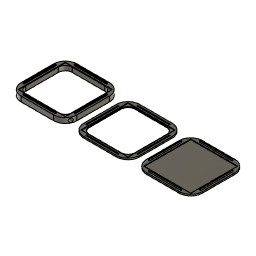
Abyssal_Mirror (Autodesk Fusion 360 design; units mm, degrees)
Autodesk Fusion 360 part; units mm, degrees
sketch "草图1" plane through (0, 0, 0) normal (0, 0, 1) x (1, 0, 0)
  line L0 (-50.5, 50.5) -> (50.5, 50.5)
  line L1 (50.5, 50.5) -> (50.5, -50.5)
  line L2 (50.5, -50.5) -> (-50.5, -50.5)
  line L3 (-50.5, -50.5) -> (-50.5, 50.5)
  line L4 (-35, 50) -> (35, 50)
  line L5 (50, 35) -> (50, -35)
  line L6 (35, -50) -> (-35, -50)
  line L7 (-50, -35) -> (-50, 35)
  arc A0 (-35, 50) -> (-50, 35) centre (-35, 35) ccw
  arc A1 (50, 35) -> (35, 50) centre (35, 35) ccw
  arc A2 (35, -50) -> (50, -35) centre (35, -35) ccw
  arc A3 (-50, -35) -> (-35, -50) centre (-35, -35) ccw
  line L8 (-35, 60) -> (35, 60)
  line L9 (60, 35) -> (60, -35)
  line L10 (35, -60) -> (-35, -60)
  line L11 (-60, -35) -> (-60, 35)
  arc A4 (60, 35) -> (35, 60) centre (35, 35) ccw
  arc A5 (-35, 60) -> (-60, 35) centre (-35, 35) ccw
  arc A6 (-60, -35) -> (-35, -60) centre (-35, -35) ccw
  arc A7 (35, -60) -> (60, -35) centre (35, -35) ccw
  dimension "d1" = 101
  dimension "d2" = 101
  dimension "d3" = 15
  dimension "d4" = 15
  dimension "d5" = 25
  constraint horizontal L0
  constraint vertical L1
  constraint horizontal L2
  constraint vertical L3
  constraint horizontal L4
  constraint vertical L5
  constraint horizontal L6
  constraint vertical L7
  constraint tangent L4 A0
  constraint tangent L7 A0
  constraint tangent L4 A1
  constraint tangent L5 A1
  constraint tangent L5 A2
  constraint tangent L6 A2
  constraint equal A1 A2
  constraint tangent L7 A3
  constraint tangent L6 A3
  constraint equal A1 A3
  constraint horizontal L8
  constraint vertical L9
  constraint horizontal L10
  constraint vertical L11
  constraint tangent L9 A4
  constraint tangent L8 A4
  constraint tangent L8 A5
  constraint tangent L11 A5
  constraint equal A4 A5
  constraint tangent L11 A6
  constraint tangent L10 A6
  constraint equal A4 A6
  constraint tangent L9 A7
  constraint tangent L10 A7
  constraint equal A4 A7
  measures "d1" distance of L0.start L0.end
  measures "d2" distance of L0.start L2.end
  measures "d3" radius of A0
  measures "d4" radius of A1
  measures "d5" radius of A4
extrude "拉伸1" add sketch "草图1" along normal blind 11 contours L8 L9 L10 L11 A4 A5 A6 A7 makes body 1
extrude "拉伸2" add sketch "草图1" along normal blind 9 contours L0 L1 L2 L3 bodies 1
sketch "草图2" plane through (0, 0, 0) normal (0, 0, 1) x (1, 0, 0)
  line L0 (-35, 56) -> (35, 56)
  line L1 (35, 56) -> (35, 54)
  line L2 (35, 54) -> (-35, 54)
  line L3 (-35, 54) -> (-35, 56)
  line L4 (53.9983, 35) -> (56, 35)
  line L5 (56, 35) -> (56, -35)
  line L6 (56, -35) -> (53.9983, -35)
  line L7 (53.9983, -35) -> (53.9983, 35)
  line L8 (-5, 0) -> (5, 0)
  line L9 (0, 5) -> (0, -5)
  line L10 (35, -56) -> (35, -54)
  line L11 (-35, -54) -> (-35, -56)
  line L12 (-35, -56) -> (35, -56)
  line L13 (35, -54) -> (-35, -54)
  line L14 (-56, -35) -> (-53.9983, -35)
  line L15 (-56, 35) -> (-56, -35)
  line L16 (-53.9983, -35) -> (-53.9983, 35)
  line L17 (-53.9983, 35) -> (-56, 35)
  constraint horizontal L0
  constraint vertical L1
  constraint horizontal L2
  constraint vertical L3
  constraint horizontal L4
  constraint vertical L5
  constraint horizontal L6
  constraint vertical L7
  constraint horizontal L8
  constraint vertical L9
  constraint symmetric L0.start L8 L11.end
  constraint symmetric L0.end L8 L10.start
  constraint symmetric L1.end L8 L10.end
  constraint symmetric L2.end L8 L11.start
  constraint symmetric L4.start L9 L16.end
  constraint symmetric L4.end L9 L15.start
  constraint symmetric L5.end L9 L14.start
  constraint symmetric L6.end L9 L14.end
extrude "拉伸3" cut sketch "草图2" along normal blind 15 bodies 1
extrude "拉伸4" add sketch "草图2" along normal blind 15 bodies 1
extrude "拉伸5" cut sketch "草图2" along normal blind 5 bodies 1
sketch "草图3" plane through (60, 0, 0) normal (1, 0, 0) x (0, 1, 0)
  line L0 (-35, 0) -> (35, 0)
  line L1 (35, 0) -> (35, 11)
  line L2 (35, 11) -> (-35, 11)
  line L3 (-35, 11) -> (-35, 0)
  circle A0 centre (-45.5, 5) radius 4
  dimension "d16" = 8
  measures "d16" diameter of A0
extrude "拉伸6" cut sketch "草图3" against normal blind 34 contours A0 bodies 1
move_body "移动1" bodies 1 to x (1, 0, 0) y (0, 1, 0) z (0, 0, 1) at (-135, 0, 0)
sketch "草图5" plane through (0, 0, 0) normal (0, 0, 1) x (1, 0, 0)
  line L0 (-34, 49) -> (34, 49)
  line L1 (49, 34) -> (49, -34)
  line L2 (34, -49) -> (-34, -49)
  line L3 (-49, -34) -> (-49, 34)
  arc A0 (-34, 49) -> (-49, 34) centre (-34, 34) ccw
  arc A1 (49, 34) -> (34, 49) centre (34, 34) ccw
  arc A2 (34, -49) -> (49, -34) centre (34, -34) ccw
  arc A3 (-49, -34) -> (-34, -49) centre (-34, -34) ccw
  dimension "d19" = 15
  constraint horizontal L0
  constraint vertical L1
  constraint horizontal L2
  constraint vertical L3
  constraint tangent L0 A0
  constraint tangent L3 A0
  constraint tangent L0 A1
  constraint tangent L1 A1
  constraint equal A0 A1
  constraint tangent L1 A2
  constraint tangent L2 A2
  constraint equal A0 A2
  constraint tangent L2 A3
  constraint tangent L3 A3
  constraint equal A0 A3
  measures "d19" radius of A0
extrude "拉伸7" add sketch "草图1" along normal blind 2 separate body contours L8 L9 L10 L11 A4 A5 A6 A7 makes body 2
extrude "拉伸8" cut 4 faces at (-146.6667, 55.3333, 15) (-190.3328, -11.6667, 15) (-80.3345, -11.6667, 15) (-123.3333, -55.3333, 15) along direction (0, 0, -1) blind 3 on bodies 1 bodies 1
extrude "拉伸9" add 4 faces at (-190.3328, -11.6667, 12) (-146.6667, 55.3333, 12) (-80.3345, -11.6667, 12) (-123.3333, -55.3333, 12) along direction (0, 0, 1) blind 1 on bodies 1 bodies 1
extrude "拉伸10" add 4 faces at (-190.3328, -11.6667, 5) (-123.3333, -55.3333, 5) (-80.3345, -11.6667, 5) (-146.6667, 55.3333, 5) along direction (0, 0, -1) blind 2 on bodies 1 bodies 1
extrude "拉伸11" add 1 faces at (-53.6667, 11.6667, 2) along direction (0, 0, 1) blind 1 on bodies 2 bodies 2
extrude "拉伸12" cut sketch "草图2" along normal blind 6 bodies 2
extrude "拉伸13" add sketch "草图2" along normal blind 6 bodies 2
extrude "拉伸14" add sketch "草图1" along normal blind 0.8 contours L0 L1 L2 L3 | L4 L5 L6 L7 A0 A1 A2 A3 bodies 2
move_body "移动2" bodies 2 to x (1, 0, 0) y (0, 1, 0) z (0, 0, 1) at (135, 0, 0)
extrude "拉伸15" add sketch "草图1" along normal blind 3 separate body contours L8 L9 L10 L11 A4 A5 A6 A7 makes body 3
extrude "拉伸16" cut sketch "草图2" along normal blind 3 bodies 3
extrude "拉伸17" add sketch "草图1" along normal blind 1.2 contours L0 L1 L2 L3 | L4 L5 L6 L7 A0 A1 A2 A3 bodies 3
extrude "拉伸18" cut sketch "草图5" along normal blind 9 bodies 3
extrude "拉伸19" add 1 faces at (-182.47, -47.47, 9) along direction (0, 0, 1) blind 1 on bodies 1 bodies 1
extrude "拉伸20" add 1 faces at (46.5531, -46.5531, 1.2) along direction (0, 0, 1) blind 1 on bodies 3 bodies 3
extrude "拉伸21" cut 1 faces at (46.5531, -46.5531, 2.2) along direction (0, 0, -1) blind 0.2 on bodies 3 bodies 3
extrude "拉伸22" add 1 faces at (118.1667, 16.8333, 0.8) along direction (0, 0, 1) blind 1 on bodies 2 bodies 2
